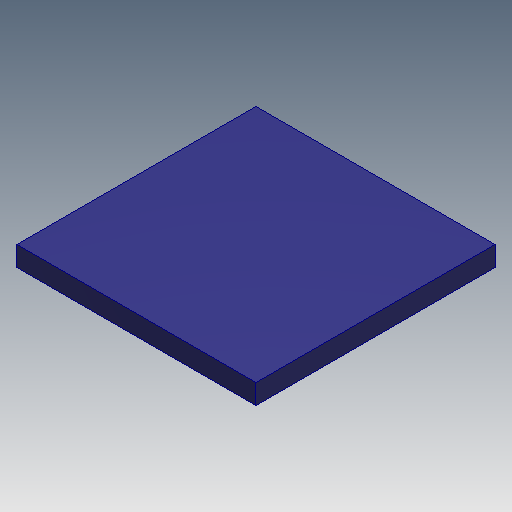
# Autodesk Inventor part: BUZZER
Saved by Autodesk Inventor 2017 (Build 210142000, 142)
## iProperties
Part Number: BUZZER
Material: Generisch
Document SubType Name: Modeling
Designer: Werkstatt
Density: 1 g/cm^3
Appearance: BUZZER-12MM, BUZZER
Author: Werkstatt
Autodesk Inventor part; units mm, degrees
ref_plane "YZ Plane" through (0, 0, 0) normal (1, 0, 0) x (0, 1, 0)
ref_plane "XZ Plane" through (0, 0, 0) normal (0, 1, 0) x (-1, 0, 0)
ref_plane "XY Plane" through (0, 0, 0) normal (0, 0, 1) x (1, 0, 0)
sketch "BUZZER-12MM, BUZZER_1" plane through (0, 0, 0) normal (0, 0, 1) x (1, 0, 0)
  line L0 (-6.0016, 6.0016) -> (6.0016, 6.0016)
  line L1 (6.0016, 6.0016) -> (6.0016, -6.0016)
  line L2 (6.0016, -6.0016) -> (-6.0016, -6.0016)
  line L3 (-6.0016, -6.0016) -> (-6.0016, 6.0016)
  constraints: 8 end point
extrude "Extrusion1" add sketch "BUZZER-12MM, BUZZER_1" along normal blind 1
